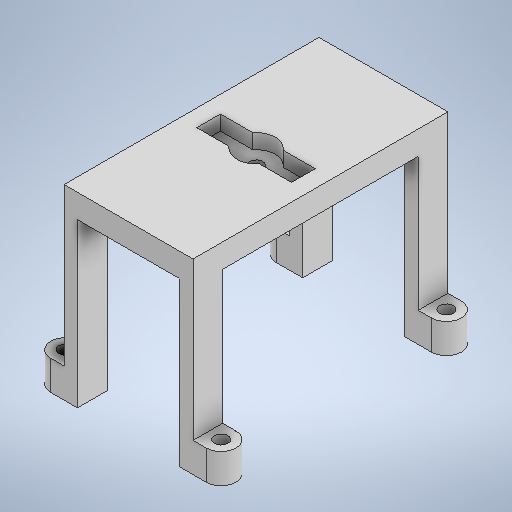
# Autodesk Inventor part: ATTACHMENT_TOOLHEAD_GRIPPER
Saved by Autodesk Inventor 2025.1 (Build 291241000, 241)
## iProperties
Created: 2024-10-27
Part Number: ATTACHMENT_TOOLHEAD_GRIPPER
Material: Generic
Document SubType Name: Modeling
Designer: m_kni
Density: 1 g/cm^3
Appearance: Default
Author: m_kni
Autodesk Inventor part; units mm, degrees
ref_plane "YZ Plane" through (0, 0, 0) normal (1, 0, 0) x (0, 1, 0)
ref_plane "XZ Plane" through (0, 0, 0) normal (0, 1, 0) x (-1, 0, 0)
ref_plane "XY Plane" through (0, 0, 0) normal (0, 0, 1) x (1, 0, 0)
sketch "Sketch1" plane through (0, 0, 0) normal (0, 1, 0) x (-1, 0, 0)
  circle A0 centre (-27.7235, -39.6791) radius 2.3
  line L0 (24.7765, 36.3209) -> (-27.7235, -39.6791)
  circle A1 centre (24.7765, -39.6791) radius 2.3
  circle A2 centre (-27.7235, 36.3209) radius 2.3
  line L1 (24.7765, -39.6791) -> (-27.7235, 36.3209)
  circle A3 centre (24.7765, 36.3209) radius 2.3
  circle A4 centre (24.7765, 36.3209) radius 2.3
  circle A5 centre (-27.7235, 36.3209) radius 2.3
  circle A6 centre (24.7765, -39.6791) radius 2.3
  circle A7 centre (-27.7235, -39.6791) radius 2.3
  circle A8 centre (-1.4735, -1.6791) radius 6.8323
  circle A9 centre (-27.7235, 36.3209) radius 5
  circle A10 centre (-27.7235, -39.6791) radius 5
  circle A11 centre (24.7765, -39.6791) radius 5
  circle A12 centre (24.7765, 36.3209) radius 5
  line L2 (-27.7235, 41.3209) -> (-18.7235, 41.3209)
  line L3 (-18.7235, 41.3209) -> (-18.7235, 31.3209)
  line L4 (-18.7235, 31.3209) -> (-27.7235, 31.3209)
  line L5 (24.7765, 41.3209) -> (15.7765, 41.3209)
  line L6 (15.7765, 41.3209) -> (15.7765, 31.3209)
  line L7 (15.7765, 31.3209) -> (24.7765, 31.3209)
  line L8 (24.7765, -34.6791) -> (15.7765, -34.6791)
  line L9 (15.7765, -34.6791) -> (15.7765, -44.6791)
  line L10 (15.7765, -44.6791) -> (24.7765, -44.6791)
  line L11 (-27.7235, -34.6791) -> (-18.7235, -34.6791)
  line L12 (-18.7235, -34.6791) -> (-18.7235, -44.6791)
  line L13 (-18.7235, -44.6791) -> (-27.7235, -44.6791)
  point P0 (0, 0)
  dimension "d0" = 10
  dimension "d1" = 10
  dimension "d2" = 10
  dimension "d3" = 10
  dimension "d4" = 9
  dimension "d5" = 9
  constraints: 28 end point, 13 centre point, 8 point on circle, 7 point on line, 7 tangent, 6 coincident, 3 concentric, 3 perpendicular, 2 horizontal, 1 midpoint, 1 parallel
  measures "d0" diameter of A9
  measures "d1" diameter of A10
  measures "d2" diameter of A11
  measures "d3" diameter of A12
  measures "d4" distance of L2.start L2.end
  measures "d5" distance of L5.start L5.end
extrude "Extrusion1" add sketch "Sketch1" along normal blind 10 contours A12 L7 L0 | L0 L7 L6 L5 A12 | A12 | L11 L12 L13 A10 L0 | L0 A10 L11 | A10 | A11 L10 L9 L8 L1 | L1 L8 A11 | A11 | L4 A9 L1 | L1 A9 L2 L3 L4 | A9
sketch "Sketch2" plane through (0, 10, 0) normal (0, 1, 0) x (1, 0, 0)
  line L0 (-15.7765, -41.3209) -> (-15.7765, -31.3209) projected
  line L1 (-15.7765, -31.3209) -> (-24.7765, -31.3209) projected
  line L2 (-15.7765, -41.3209) -> (-20.2765, -41.3209)
  line L3 (-20.2765, -41.3209) -> (-20.2765, -31.3209)
  line L4 (-20.2765, -31.3209) -> (-15.7765, -31.3209)
  line L5 (-15.7765, -31.3209) -> (-15.7765, -41.3209)
  line L6 (-24.7765, 34.6791) -> (-15.7765, 34.6791) projected
  line L7 (-15.7765, 44.6791) -> (-24.7765, 44.6791) projected
  line L8 (-15.7765, 34.6791) -> (-20.2765, 34.6791)
  line L9 (-20.2765, 34.6791) -> (-20.2765, 44.6791)
  line L10 (-20.2765, 44.6791) -> (-15.7765, 44.6791)
  line L11 (-15.7765, 44.6791) -> (-15.7765, 34.6791)
  line L12 (18.7235, 34.6791) -> (23.2235, 34.6791)
  line L13 (23.2235, 34.6791) -> (23.2235, 44.6791)
  line L14 (23.2235, 44.6791) -> (18.7235, 44.6791)
  line L15 (18.7235, 44.6791) -> (18.7235, 34.6791)
  line L16 (18.7235, -41.3209) -> (27.7235, -41.3209) projected
  line L17 (18.7235, -41.3209) -> (23.2235, -41.3209)
  line L18 (23.2235, -41.3209) -> (23.2235, -31.3209)
  line L19 (23.2235, -31.3209) -> (18.7235, -31.3209)
  line L20 (18.7235, -31.3209) -> (18.7235, -41.3209)
  point P0 (0, 0)
  constraints: 32 end point, 8 parallel, 4 horizontal, 4 perpendicular, 2 midpoint, 2 point on line
extrude "Extrusion2" add sketch "Sketch2" along normal blind 45
sketch "Sketch3" plane through (0, 55, 0) normal (0, 1, 0) x (1, 0, 0)
  line L0 (-20.2765, -41.3209) -> (-20.2765, -31.3209) projected
  line L1 (27.7235, 44.6791) -> (18.7235, 44.6791) projected
  line L2 (-20.2765, -41.3209) -> (23.2235, -41.3209)
  line L3 (23.2235, -41.3209) -> (23.2235, 44.6791)
  line L4 (23.2235, 44.6791) -> (-20.2765, 44.6791)
  line L5 (-20.2765, 44.6791) -> (-20.2765, -41.3209)
  point P0 (0, 0)
  constraints: 8 end point, 2 parallel, 1 horizontal, 1 midpoint, 1 perpendicular
extrude "Extrusion3" add sketch "Sketch3" along normal blind 8
sketch "Sketch4" plane through (0, 63, 0) normal (0, 1, 0) x (1, 0, 0)
  line L0 (-20.2765, 44.6791) -> (-20.2765, -41.3209) projected
  line L1 (-20.2765, -41.3209) -> (23.4801, 44.6791)
  line L2 (23.2235, -41.3209) -> (23.2235, 44.6791) projected
  line L3 (23.2235, 44.6791) -> (-20.2765, 44.6791) projected
  line L4 (23.2235, -41.3209) -> (-20.2765, 44.6791)
  circle A0 centre (1.4735, 1.6791) radius 6.5
  line L5 (17.4735, 5.6791) -> (-14.5265, 5.6791)
  line L6 (-14.5265, 5.6791) -> (-14.5265, -2.3209)
  line L7 (-14.5265, -2.3209) -> (17.4735, -2.3209)
  line L8 (17.4735, -2.3209) -> (17.4735, 5.6791)
  line L9 (17.4735, 5.6791) -> (-14.5265, -2.3209) construction
  line L10 (-14.5265, 5.6791) -> (17.4735, -2.3209) construction
  point P0 (0, 0)
  point P1 (-3.65, 5.6791)
  point P2 (-3.65, -2.3209)
  point P3 (6.597, -2.3209)
  point P4 (6.597, 5.6791)
  dimension "d13" = 13
  dimension "d14" = 32
  dimension "d15" = 8
  constraints: 16 end point, 3 midpoint, 2 parallel, 1 centre point, 1 horizontal, 1 perpendicular
  measures "d13" diameter of A0
  measures "d14" distance of L7.end L6.end
  measures "d15" distance of L6.end L5.end
extrude "Extrusion4" cut sketch "Sketch4" against normal blind 5 contours A0 L1 L5 L4 | L4 L5 A0 | A0 L7 L1 | L1 L7 L4 A0 | L5 L1 L4 | L4 L1 L7 A0 L5 | A0 L5 L1 | A0 L7 L6 L5 | L1 L4 L7 | L4 L7 A0 | L1 L5 A0 L7 L4 | L5 L8 L7 A0
sketch "Sketch5" plane through (0, 58, 0) normal (0, 1, 0) x (1, 0, 0)
  arc A0 (6.597, 5.6791) -> (-3.65, 5.6791) centre (1.4735, 1.6791) ccw projected
  arc A1 (-3.65, -2.3209) -> (6.597, -2.3209) centre (1.4735, 1.6791) ccw projected
  circle A2 centre (1.4735, 1.6791) radius 2.25
  point P0 (0, 0)
  dimension "d18" = 4.5
  constraints: 1 centre point, 1 coincident
  measures "d18" diameter of A2
extrude "Extrusion5" cut sketch "Sketch5" against normal blind 8
body "Solid1"
